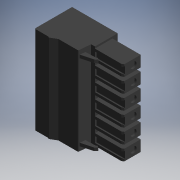
# Autodesk Inventor part: 5065802 6GD-1RR7.62-CLP-CBL
Saved by Autodesk Inventor 2017.3 (Build 213256000, 256)
## iProperties
Part Number: 5065802 6GD-1RR7.62-CLP-CBL
Material: Generic
Catalog Web Link: www.cadenas.de
Description: NEKM-C6 (p)-Terminal strip
Vendor: FESTO
Document SubType Name: Modeling
Designer: partserver
Manufacturer: FESTO
Mass: 21.6186 g
Surface Area: 92.1465 cm^2
Volume: 21.6186 cm^3
Density: 1 g/cm^3
Appearance: PSOLRGB-80-80-80
Category: PARTsolutions
Company: FESTO
Title: 5065802 6GD-1RR7.62-CLP-CBL
Author: Cadenas PARTsolutions
Comments: Terminal strip
PSOL_IDENT_0: {$CADENAS_DATA\23d-libs\festo\parts\n\nekm\parts\nekm_c6_parts.prj},199 {VTYP=3D},{NB=5065802 6GD-1R
PSOL_IDENT_1: R7.62-CLP-CBL},{LINA=5065802 6GD-1RR7.62-CLP-CBL},{NN=NEKM-C6 (p)},{DATE=16.05.2019 05:36:58},{GEOMD
PSOL_IDENT_2: ATE=16.05.2019 05:36:56},{VERSION=},{LINEID=90},{WBVAR=},{WBNUMERIC=}  {NB=5065802 6GD-1RR7.62-CLP-C
PSOL_IDENT_3: BL},{LINA=5065802 6GD-1RR7.62-CLP-CBL},{KT=DUMMY},{TNR=5065802},{TYP=6GD-1RR7.62-CLP-CBL},{VERS=5},{
PSOL_IDENT_4: N=6},{L=45.720},{L1=0.000}
NB: 5065802 6GD-1RR7.62-CLP-CBL
NN: NEKM-C6 (p)
NT: Terminal strip
NBSYN: $TNR. $TYP.
LINA: 5065802 6GD-1RR7.62-CLP-CBL
CATALOG: Festo
TNR: 5065802
TYP: 6GD-1RR7.62-CLP-CBL
VERS: 5
N: 6
L: 45.72
L1: 0
SUPPLIER: FESTO
ARTICLENO: 5065802 6GD-1RR7.62-CLP-CBL
BOMINFO: 5065802 6GD-1RR7.62-CLP-CBL
CREATOR: CADENAS GmbH
Autodesk Inventor part; units mm, degrees
ref_plane "YZ Plane" through (0, 0, 0) normal (1, 0, 0) x (0, 1, 0)
ref_plane "XZ Plane" through (0, 0, 0) normal (0, 1, 0) x (-1, 0, 0)
ref_plane "XY Plane" through (0, 0, 0) normal (0, 0, 1) x (1, 0, 0)
sketch "Sketch_14" plane through (0, 0, 0) normal (0, 0, 1) x (1, 0, 0)
  line L0 (-14.7, -1.3876) -> (-13.7, -1.965)
  line L1 (-13.7, -1.965) -> (2, -1.965)
  line L2 (2, -1.965) -> (2.4968, -7.6436)
  arc A0 (2.4968, -7.6436) -> (2.9949, -8.1) centre (2.9949, -7.6) ccw
  line L3 (2.9949, -8.1) -> (12.85, -8.1)
  line L4 (12.85, -8.1) -> (15.9677, -9.9)
  line L5 (15.9677, -9.9) -> (16.25, -9.9)
  arc A1 (16.25, -9.9) -> (16.45, -9.7) centre (16.25, -9.7) ccw
  line L6 (16.45, -9.7) -> (16.45, -9.6)
  line L7 (16.45, -9.6) -> (23.25, -9.6)
  arc A2 (23.25, -9.6) -> (23.75, -9.1) centre (23.25, -9.1) ccw
  line L8 (23.75, -9.1) -> (23.75, 9.9)
  line L9 (23.75, 9.9) -> (-14.7, 9.9)
  line L10 (-14.7, 9.9) -> (-14.7, -1.3876)
  constraints: 22 end point, 6 point on circle, 3 centre point
extrude "Extrusion1" add sketch "Sketch_14" along normal mid plane 45.72
sketch "Sketch_4" plane through (25.8, 0, 0) normal (1, 0, 0) x (0, 0, -1)
  line L0 (-22.26, 6.0143) -> (-22.26, 3.1857)
  arc A0 (-22.26, 3.1857) -> (-15.84, 3.1857) centre (-19.05, 4.45) ccw
  line L1 (-15.84, 3.1857) -> (-15.84, 6.0143)
  arc A1 (-15.84, 6.0143) -> (-22.26, 6.0143) centre (-19.05, 4.75) ccw
  constraints: 4 end point, 4 point on circle, 2 centre point
extrude "Extrusion2" cut sketch "Sketch_4" against normal blind 10
pattern_linear "Rectangular Pattern1" count 6 spacing 7.62 along (0, 0, -1) of "Extrusion2"
sketch "Sketch_6" plane through (25.8, 0, 0) normal (1, 0, 0) x (0, 0, -1)
  line L0 (-20.9, -4.05) -> (-17.2, -4.05)
  line L1 (-17.2, -4.05) -> (-17.2, -0.2)
  line L2 (-17.2, -0.2) -> (-20.9, -0.2)
  line L3 (-20.9, -0.2) -> (-20.9, -4.05)
  constraints: 8 end point
extrude "Extrusion3" cut sketch "Sketch_6" against normal blind 7
pattern_linear "Rectangular Pattern2" count 6 spacing 7.62 along (0, 0, -1) of "Extrusion3"
sketch "Sketch_15" plane through (-14.7, 0, 0) normal (1, 0, 0) x (0, 0, -1)
  line L0 (-22.86, -3.965) -> (22.86, -3.965)
  line L1 (22.86, -3.965) -> (22.86, 9.9)
  line L2 (22.86, 9.9) -> (-22.86, 9.9)
  line L3 (-22.86, 9.9) -> (-22.86, -3.965)
  line L4 (16.2, -1.965) -> (17.53, -1.965)
  line L5 (17.53, -1.965) -> (17.53, -1.7722)
  arc A0 (17.53, -1.7722) -> (17.4847, -1.6479) centre (17.3365, -1.7722) ccw
  line L6 (17.4847, -1.6479) -> (17.2448, -1.3619)
  arc A1 (17.393, -1.044) -> (17.2448, -1.3619) centre (17.393, -1.2375) ccw
  line L7 (17.393, -1.044) -> (20.707, -1.044)
  arc A2 (20.8552, -1.3619) -> (20.707, -1.044) centre (20.707, -1.2375) ccw
  line L8 (20.8552, -1.3619) -> (20.6153, -1.6479)
  arc A3 (20.6153, -1.6479) -> (20.57, -1.7722) centre (20.7635, -1.7722) ccw
  line L9 (20.57, -1.7722) -> (20.57, -1.965)
  line L10 (20.57, -1.965) -> (21.9, -1.965)
  line L11 (21.9, -1.965) -> (21.9, 7.165)
  line L12 (21.9, 7.165) -> (16.2, 7.165)
  line L13 (16.2, 7.165) -> (16.2, -1.965)
  line L14 (8.58, -1.965) -> (9.91, -1.965)
  line L15 (9.91, -1.965) -> (9.91, -1.7722)
  arc A4 (9.91, -1.7722) -> (9.8647, -1.6479) centre (9.7165, -1.7722) ccw
  line L16 (9.8647, -1.6479) -> (9.6248, -1.3619)
  arc A5 (9.773, -1.044) -> (9.6248, -1.3619) centre (9.773, -1.2375) ccw
  line L17 (9.773, -1.044) -> (13.087, -1.044)
  arc A6 (13.2352, -1.3619) -> (13.087, -1.044) centre (13.087, -1.2375) ccw
  line L18 (13.2352, -1.3619) -> (12.9953, -1.6479)
  arc A7 (12.9953, -1.6479) -> (12.95, -1.7722) centre (13.1435, -1.7722) ccw
  line L19 (12.95, -1.7722) -> (12.95, -1.965)
  line L20 (12.95, -1.965) -> (14.28, -1.965)
  line L21 (14.28, -1.965) -> (14.28, 7.165)
  line L22 (14.28, 7.165) -> (8.58, 7.165)
  line L23 (8.58, 7.165) -> (8.58, -1.965)
  line L24 (0.96, -1.965) -> (2.29, -1.965)
  line L25 (2.29, -1.965) -> (2.29, -1.7722)
  arc A8 (2.29, -1.7722) -> (2.2447, -1.6479) centre (2.0965, -1.7722) ccw
  line L26 (2.2447, -1.6479) -> (2.0048, -1.3619)
  arc A9 (2.153, -1.044) -> (2.0048, -1.3619) centre (2.153, -1.2375) ccw
  line L27 (2.153, -1.044) -> (5.467, -1.044)
  arc A10 (5.6152, -1.3619) -> (5.467, -1.044) centre (5.467, -1.2375) ccw
  line L28 (5.6152, -1.3619) -> (5.3753, -1.6479)
  arc A11 (5.3753, -1.6479) -> (5.33, -1.7722) centre (5.5235, -1.7722) ccw
  line L29 (5.33, -1.7722) -> (5.33, -1.965)
  line L30 (5.33, -1.965) -> (6.66, -1.965)
  line L31 (6.66, -1.965) -> (6.66, 7.165)
  line L32 (6.66, 7.165) -> (0.96, 7.165)
  line L33 (0.96, 7.165) -> (0.96, -1.965)
  line L34 (-6.66, -1.965) -> (-5.33, -1.965)
  line L35 (-5.33, -1.965) -> (-5.33, -1.7722)
  arc A12 (-5.33, -1.7722) -> (-5.3753, -1.6479) centre (-5.5235, -1.7722) ccw
  line L36 (-5.3753, -1.6479) -> (-5.6152, -1.3619)
  arc A13 (-5.467, -1.044) -> (-5.6152, -1.3619) centre (-5.467, -1.2375) ccw
  line L37 (-5.467, -1.044) -> (-2.153, -1.044)
  arc A14 (-2.0048, -1.3619) -> (-2.153, -1.044) centre (-2.153, -1.2375) ccw
  line L38 (-2.0048, -1.3619) -> (-2.2447, -1.6479)
  arc A15 (-2.2447, -1.6479) -> (-2.29, -1.7722) centre (-2.0965, -1.7722) ccw
  line L39 (-2.29, -1.7722) -> (-2.29, -1.965)
  line L40 (-2.29, -1.965) -> (-0.96, -1.965)
  line L41 (-0.96, -1.965) -> (-0.96, 7.165)
  line L42 (-0.96, 7.165) -> (-6.66, 7.165)
  line L43 (-6.66, 7.165) -> (-6.66, -1.965)
  line L44 (-14.28, -1.965) -> (-12.95, -1.965)
  line L45 (-12.95, -1.965) -> (-12.95, -1.7722)
  arc A16 (-12.95, -1.7722) -> (-12.9953, -1.6479) centre (-13.1435, -1.7722) ccw
  line L46 (-12.9953, -1.6479) -> (-13.2352, -1.3619)
  arc A17 (-13.087, -1.044) -> (-13.2352, -1.3619) centre (-13.087, -1.2375) ccw
  line L47 (-13.087, -1.044) -> (-9.773, -1.044)
  arc A18 (-9.6248, -1.3619) -> (-9.773, -1.044) centre (-9.773, -1.2375) ccw
  line L48 (-9.6248, -1.3619) -> (-9.8647, -1.6479)
  arc A19 (-9.8647, -1.6479) -> (-9.91, -1.7722) centre (-9.7165, -1.7722) ccw
  line L49 (-9.91, -1.7722) -> (-9.91, -1.965)
  line L50 (-9.91, -1.965) -> (-8.58, -1.965)
  line L51 (-8.58, -1.965) -> (-8.58, 7.165)
  line L52 (-8.58, 7.165) -> (-14.28, 7.165)
  line L53 (-14.28, 7.165) -> (-14.28, -1.965)
  line L54 (-21.9, 7.165) -> (-21.9, -1.965)
  line L55 (-21.9, -1.965) -> (-20.57, -1.965)
  line L56 (-20.57, -1.965) -> (-20.57, -1.7722)
  arc A20 (-20.57, -1.7722) -> (-20.6153, -1.6479) centre (-20.7635, -1.7722) ccw
  line L57 (-20.6153, -1.6479) -> (-20.8552, -1.3619)
  arc A21 (-20.707, -1.044) -> (-20.8552, -1.3619) centre (-20.707, -1.2375) ccw
  line L58 (-20.707, -1.044) -> (-17.393, -1.044)
  arc A22 (-17.2448, -1.3619) -> (-17.393, -1.044) centre (-17.393, -1.2375) ccw
  line L59 (-17.2448, -1.3619) -> (-17.4847, -1.6479)
  arc A23 (-17.4847, -1.6479) -> (-17.53, -1.7722) centre (-17.3365, -1.7722) ccw
  line L60 (-17.53, -1.7722) -> (-17.53, -1.965)
  line L61 (-17.53, -1.965) -> (-16.2, -1.965)
  line L62 (-16.2, -1.965) -> (-16.2, 7.165)
  line L63 (-16.2, 7.165) -> (-21.9, 7.165)
  constraints: 128 end point, 48 point on circle, 24 centre point
extrude "Extrusion4" cut sketch "Sketch_15" along normal blind 14.7
sketch "Sketch5" plane through (-14.7, -1.3876, 21.9) normal (-1, 0, 0) x (0, 0, 1)
  point P0 (-2.85, 4.7876)
hole "Hole1" at (-14.7, 3.4, 19.05) direction (1, 0, 0) diameter 3.2 depth 1
pattern_linear "Rectangular Pattern3" count 6 spacing 7.62 along (0, 0, -1) of "Hole1"
sketch "Sketch_18" plane through (0, 0, 20.65) normal (0, 0, 1) x (1, 0, 0)
  arc A0 (-4.3591, -4.5663) -> (-4.4005, -4.881) centre (-4.2591, -4.7395) ccw
  line L0 (-4.4005, -4.881) -> (-3.6104, -5.6711)
  arc A1 (-3.6104, -5.6711) -> (-3.2742, -5.8652) centre (-3.08, -5.1408) ccw
  line L1 (-3.2742, -5.8652) -> (2.476, -7.406)
  line L2 (2.476, -7.406) -> (2.2406, -4.715)
  line L3 (2.2406, -4.715) -> (-3.03, -4.4849)
  line L4 (-3.03, -4.4849) -> (-3.3021, -4.2128)
  arc A2 (-3.3021, -4.2128) -> (-3.6642, -4.1651) centre (-3.5142, -4.4249) ccw
  line L5 (-3.6642, -4.1651) -> (-4.3591, -4.5663)
  constraints: 12 end point, 6 point on circle, 3 centre point
extrude "Extrusion5" add sketch "Sketch_18" against normal blind 1.6
sketch "Sketch_19" plane through (0, 0, -20.65) normal (0, 0, 1) x (1, 0, 0)
  arc A0 (-4.3591, -4.5663) -> (-4.4005, -4.881) centre (-4.2591, -4.7395) ccw
  line L0 (-4.4005, -4.881) -> (-3.6104, -5.6711)
  arc A1 (-3.6104, -5.6711) -> (-3.2742, -5.8652) centre (-3.08, -5.1408) ccw
  line L1 (-3.2742, -5.8652) -> (2.476, -7.406)
  line L2 (2.476, -7.406) -> (2.2406, -4.715)
  line L3 (2.2406, -4.715) -> (-3.03, -4.4849)
  line L4 (-3.03, -4.4849) -> (-3.3021, -4.2128)
  arc A2 (-3.3021, -4.2128) -> (-3.6642, -4.1651) centre (-3.5142, -4.4249) ccw
  line L5 (-3.6642, -4.1651) -> (-4.3591, -4.5663)
  constraints: 12 end point, 6 point on circle, 3 centre point
extrude "Extrusion6" add sketch "Sketch_19" along normal blind 1.6
ref_plane "ANBAU_XY" through (0, 0, 0) normal (0, 1, 0) x (1, 0, 0)
ref_plane "ANBAU_YZ" through (0, 0, 0) normal (1, 0, 0) x (0, 0, -1)
ref_plane "ANBAU_ZX" through (0, 0, 0) normal (0, 0, -1) x (0, 1, 0)
body "Solid1"
